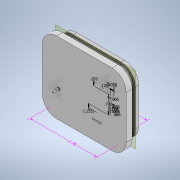
# Autodesk Inventor part: Top_Housing_K30_Elipse_O_Ring
Saved by Autodesk Inventor 2022 (Build 260153000, 153)
## iProperties
Created: 2022-06-02
Part Number: Top_Housing_K30_Elipse_O_Ring
Material: Generic
Document SubType Name: Modeling
Designer: light
Density: 1 g/cm^3
Appearance: Default
Author: light
Autodesk Inventor part; units mm, degrees
ref_plane "YZ Plane" through (0, 0, 0) normal (1, 0, 0) x (0, 1, 0)
ref_plane "XZ Plane" through (0, 0, 0) normal (0, 1, 0) x (-1, 0, 0)
ref_plane "XY Plane" through (0, 0, 0) normal (0, 0, 1) x (1, 0, 0)
sketch "Sketch1" plane through (0, 0, 0) normal (0, 0, 1) x (1, 0, 0)
  line L0 (0, 0) -> (63.246, 0)
  line L1 (63.246, 0) -> (63.246, 51.689)
  line L2 (63.246, 51.689) -> (0, 51.689)
  line L3 (0, 51.689) -> (0, 0)
  dimension "d0" = 63.246
  dimension "d1" = 51.689
  constraints: 8 end point, 2 parallel, 1 horizontal, 1 perpendicular
  measures "d0" distance of L1.end L2.end
  measures "d1" distance of L0.end L1.end
extrude "Extrusion1" add sketch "Sketch1" along normal blind 10.668
sketch "Sketch2" plane through (0, 0, 10.668) normal (0, 0, 1) x (1, 0, 0)
  line L0 (61.976, 50.6053) -> (6.35, 50.6053)
  line L1 (1.27, 45.5253) -> (1.27, 17.78)
  line L2 (6.35, 12.7) -> (61.976, 12.7)
  line L3 (61.976, 12.7) -> (61.976, 50.6053)
  arc A0 (6.35, 50.6053) -> (1.27, 45.5253) centre (6.35, 45.5253) ccw
  arc A1 (1.27, 17.78) -> (6.35, 12.7) centre (6.35, 17.78) ccw
  line L4 (0, 51.689) -> (0, 0) projected
  line L5 (63.246, 0) -> (63.246, 51.689) projected
  line L6 (0, 0) -> (63.246, 0) projected
  dimension "d4" = 5.08
  dimension "d5" = 5.08
  dimension "d6" = 1.27
  dimension "d7" = 1.27
  dimension "d8" = 60.706
  dimension "d9" = 12.7
  constraints: 8 end point, 4 point on circle, 4 tangent, 2 centre point, 2 perpendicular, 1 horizontal, 1 vertical
  measures "d4" radius of A0
  measures "d5" radius of A1
  measures "d6" distance between parallel lines of L4 L1
  measures "d7" distance between parallel lines of L5 L3
  measures "d8" distance between parallel lines of L1 L3
  measures "d9" distance between parallel lines of L6 L2
extrude "Extrusion2" cut sketch "Sketch2" against normal blind 10.668
sketch "Sketch3" plane through (0, 0, 10.668) normal (0, 0, 1) x (1, 0, 0)
  line L0 (52.451, 10.2108) -> (36.957, 10.2108)
  line L1 (36.957, 10.2108) -> (36.957, 4.1148)
  line L2 (36.957, 4.1148) -> (52.451, 4.1148)
  line L3 (52.451, 4.1148) -> (52.451, 10.2108)
  line L4 (63.246, 0) -> (63.246, 51.689) projected
  line L5 (0, 0) -> (63.246, 0) projected
  dimension "d12" = 10.795
  dimension "d13" = 15.494
  dimension "d14" = 6.096
  dimension "d15" = 4.1148
  constraints: 8 end point, 2 parallel, 1 horizontal, 1 perpendicular
  measures "d12" distance between parallel lines of L4 L3
  measures "d13" distance of L1.end L2.end
  measures "d14" distance of L0.end L1.end
  measures "d15" distance between parallel lines of L5 L2
extrude "Extrusion3" cut sketch "Sketch3" against normal blind 10.668
sketch "Sketch6" plane through (0, 0, 10.668) normal (0, 0, 1) x (1, 0, 0)
  line L0 (-3.048, 55.118) -> (67.048, 55.118) projected
  line L1 (67.048, -3.048) -> (-3.048, -3.048) projected
  line L2 (67.048, 55.118) -> (-3.048, 55.118)
  line L3 (-3.048, 55.118) -> (-3.048, -3.048)
  line L4 (-3.048, -3.048) -> (67.048, -3.048)
  line L5 (67.048, -3.048) -> (67.048, 55.118)
  line L6 (61.976, 50.6053) -> (6.35, 50.6053) projected
  line L7 (6.35, 12.7) -> (61.976, 12.7) projected
  line L8 (0, 0) -> (63.246, 0) projected
  dimension "d37" = 37.9053
  dimension "d93" = 3.048
  constraints: 8 end point, 2 parallel, 1 horizontal, 1 perpendicular
  measures "d37" distance between parallel lines of L6 L7
  measures "d93" distance between parallel lines of L1 L8
extrude "Extrusion5" add sketch "Sketch6" along normal blind 6.35
sketch "Sketch8" plane through (0, 0, 10.668) normal (0, 0, -1) x (-1, 0, 0)
  line L0 (-61.5188, 13.208) -> (-42.9768, 13.208)
  line L1 (-42.9768, 13.208) -> (-42.9768, 39.878)
  line L2 (-42.9768, 39.878) -> (-61.5188, 39.878)
  line L3 (-61.5188, 39.878) -> (-61.5188, 13.208)
  line L4 (-6.35, 12.7) -> (-61.976, 12.7) projected
  line L5 (-61.976, 12.7) -> (-61.976, 50.6053) projected
  line L6 (0, 51.689) -> (0, 0) projected
  dimension "d29" = 0.508
  dimension "d30" = 0.4572
  dimension "d31" = 18.542
  dimension "d32" = 26.67
  dimension "d33" = 42.9768
  constraints: 8 end point, 2 parallel, 1 horizontal, 1 perpendicular
  measures "d29" distance between parallel lines of L4 L0
  measures "d30" distance between parallel lines of L5 L3
  measures "d31" distance of L1.end L2.end
  measures "d32" distance of L0.end L1.end
  measures "d33" distance between parallel lines of L6 L1
extrude "Extrusion7" cut sketch "Sketch8" against normal blind 4.572
fillet "Fillet1" radius 0.254 4 edges at (52.2478, 39.878, 10.668) (42.9768, 26.543, 10.668) (52.2478, 13.208, 10.668) (61.5188, 26.543, 10.668)
sketch "Sketch9" plane through (0, 0, 15.24) normal (0, 0, -1) x (-1, 0, 0)
  line L0 (-60.2488, 17.145) -> (-57.0738, 17.145)
  line L1 (-57.0738, 17.145) -> (-57.0738, 35.941)
  line L2 (-57.0738, 35.941) -> (-60.2488, 35.941)
  line L3 (-60.2488, 35.941) -> (-60.2488, 17.145)
  line L4 (-61.5188, 13.208) -> (-61.5188, 39.878) projected
  line L5 (-61.5188, 39.878) -> (-42.9768, 39.878) projected
  line L6 (-42.9768, 13.208) -> (-61.5188, 13.208) projected
  circle A0 centre (-58.6613, 24.003) radius 0.8382
  circle A1 centre (-58.6613, 26.543) radius 0.8382
  circle A2 centre (-58.6613, 29.083) radius 0.8382
  circle A3 centre (-58.6613, 21.463) radius 0.8382
  circle A4 centre (-58.6613, 34.163) radius 0.8382
  point P0 (0, 0)
  dimension "d38" = 18.796
  dimension "d39" = 1.27
  dimension "d40" = 3.175
  dimension "d41" = 3.937
  dimension "d42" = 3.937
  dimension "d114" = 1.6764
  dimension "d116" = 1.6764
  dimension "d118" = 1.6764
  dimension "d127" = 2.54
  dimension "d128" = 2.54
  dimension "d146" = 1.6764
  dimension "d148" = 2.54
  dimension "d149" = 1.6764
  constraints: 8 end point, 5 centre point, 2 parallel, 1 horizontal, 1 perpendicular
  measures "d38" distance of L0.end L1.end
  measures "d39" distance between parallel lines of L4 L3
  measures "d40" distance of L1.end L2.end
  measures "d41" distance between parallel lines of L5 L2
  measures "d42" distance between parallel lines of L6 L0
  measures "d114" diameter of A0
  measures "d116" diameter of A1
  measures "d118" diameter of A2
  measures "d127" distance of A0.centre A1.centre
  measures "d128" distance of A1.centre A2.centre
  measures "d146" diameter of A3
  measures "d148" distance of A0.centre A3.centre
  measures "d149" diameter of A4
sketch "Sketch11" plane through (0, 0, 17.018) normal (0, 0, 1) x (1, 0, 0)
  line L0 (61.976, 12.7) -> (61.976, 50.6053) projected
  line L1 (61.976, 50.6053) -> (-0.754, 50.6053)
  line L2 (-0.754, 50.6053) -> (-0.754, 12.7)
  line L3 (-0.754, 12.7) -> (61.976, 12.7)
  line L4 (61.976, 12.7) -> (61.976, 50.6053)
  circle A0 centre (56.896, 46.8013) radius 1.0033
  circle A1 centre (4.9135, 16.5958) radius 1.0033
  point P0 (0, 0)
  dimension "d59" = 2.0066
  dimension "d60" = 2.0066
  dimension "d61" = 5.08
  constraints: 8 end point, 2 centre point, 2 parallel, 1 horizontal, 1 perpendicular
  measures "d59" diameter of A0
  measures "d60" diameter of A1
  measures "d61" distance from line of L0 A0.centre
extrude "Extrusion10" add sketch "Sketch11" along normal blind 3 contours A0 | A1
sketch "Sketch12" plane through (56.896, 46.8013, 20.018) normal (0, 0, 1) x (1, 0, 0)
  circle A0 centre (0, 0) radius 1.0033 projected
  circle A1 centre (0, 0) radius 1.2446
  point P0 (-56.896, -46.8013)
  dimension "d64" = 2.4892
  constraints: 1 centre point, 1 coincident
  measures "d64" diameter of A1
sketch "Sketch13" plane through (4.9135, 16.5958, 20.018) normal (0, 0, 1) x (1, 0, 0)
  circle A0 centre (0, 0) radius 1.2446
  point P0 (-4.9135, -16.5958)
  dimension "d65" = 2.4892
  constraints: 1 centre point
  measures "d65" diameter of A0
extrude "Extrusion11" add sketch "Sketch12" along normal blind 1 contours A0 | A1
extrude "Extrusion12" add sketch "Sketch13" along normal blind 1
sketch "Sketch14" plane through (56.896, 46.8013, 21.018) normal (0, 0, 1) x (1, 0, 0)
  circle A0 centre (0, 0) radius 0.8509
  point P0 (-56.896, -46.8013)
  dimension "d70" = 1.7018
  constraints: 1 centre point
  measures "d70" diameter of A0
sketch "Sketch15" plane through (4.9135, 16.5958, 21.018) normal (0, 0, 1) x (1, 0, 0)
  circle A0 centre (0, 0) radius 1.0033 projected
  circle A1 centre (0, 0) radius 0.8509
  point P0 (-4.9135, -16.5958)
  dimension "d71" = 1.7018
  constraints: 1 centre point, 1 coincident
  measures "d71" diameter of A1
extrude "Extrusion13" add sketch "Sketch14" along normal blind 2
extrude "Extrusion14" add sketch "Sketch15" along normal blind 2 contours A1
loft "Loft1" add section 1 edges at (4.0626, 16.5958, 23.018) section 2 edges at (3.6689, 16.5958, 21.018)
loft "Loft2" add section 1 edges at (56.0451, 46.8013, 23.018) section 2 edges at (55.6514, 46.8013, 21.018)
sketch "Sketch16" plane through (56.896, 46.8013, 23.018) normal (0, 0, 1) x (1, 0, 0)
  circle A0 centre (0, 0) radius 0.7493
  point P0 (-56.896, -46.8013)
  dimension "d84" = 1.4986
  constraints: 1 centre point
  measures "d84" diameter of A0
sketch "Sketch17" plane through (4.9135, 16.5958, 23.018) normal (0, 0, 1) x (1, 0, 0)
  circle A0 centre (0, 0) radius 0.7493
  point P0 (-4.9135, -16.5958)
  dimension "d85" = 1.4986
  constraints: 1 centre point
  measures "d85" diameter of A0
extrude "Extrusion15" cut sketch "Sketch16" against normal blind 12.446
extrude "Extrusion16" cut sketch "Sketch17" against normal blind 12.446
sketch "Sketch23" plane through (-3.048, -3.048, 10.668) normal (0, -1, 0) x (1, 0, 0)
  line L0 (70.096, 0) -> (70.096, 6.35) projected
  line L1 (0, 0) -> (70.096, 0) projected
  line L2 (70.096, 6.35) -> (0, 6.35)
  line L3 (0, 6.35) -> (0, 0)
  line L4 (0, 0) -> (70.096, 0)
  line L5 (70.096, 0) -> (70.096, 6.35)
  point P0 (3.048, -10.668)
  constraints: 8 end point, 2 parallel, 1 horizontal, 1 perpendicular
extrude "Extrusion17" add sketch "Sketch23" along normal blind 0.9525
sketch "Sketch24" plane through (-3.048, 55.118, 10.668) normal (0, 1, 0) x (1, 0, 0)
  line L0 (70.096, 0) -> (70.096, -6.35) projected
  line L1 (0, 0) -> (0, -6.35) projected
  line L2 (70.096, 0) -> (0, 0)
  line L3 (0, 0) -> (0, -6.35)
  line L4 (0, -6.35) -> (70.096, -6.35)
  line L5 (70.096, -6.35) -> (70.096, 0)
  point P0 (3.048, 10.668)
  constraints: 8 end point, 2 parallel, 1 horizontal, 1 perpendicular
extrude "Extrusion18" add sketch "Sketch24" along normal blind 0.5715
sketch "Sketch25" plane through (67.048, -4.0005, 17.018) normal (1, 0, 0) x (0, 0, -1)
  line L0 (0, 0) -> (0, 59.69) projected
  line L1 (6.35, 0) -> (6.35, 59.69) projected
  line L2 (0, 0) -> (6.35, 0)
  line L3 (6.35, 0) -> (6.35, 59.69)
  line L4 (6.35, 59.69) -> (0, 59.69)
  line L5 (0, 59.69) -> (0, 0)
  point P0 (17.018, 4.0005)
  constraints: 8 end point, 2 parallel, 1 horizontal, 1 perpendicular
extrude "Extrusion19" add sketch "Sketch25" along normal blind 0.635
sketch "Sketch26" plane through (-3.048, -4.0005, 10.668) normal (-1, 0, 0) x (0, 0, 1)
  line L0 (6.35, 0) -> (0, 0) projected
  line L1 (6.35, 0) -> (6.35, 59.69) projected
  line L2 (0, 0) -> (6.35, 0)
  line L3 (6.35, 0) -> (6.35, 59.69)
  line L4 (6.35, 59.69) -> (0, 59.69)
  line L5 (0, 59.69) -> (0, 0)
  point P0 (-10.668, 4.0005)
  constraints: 8 end point, 2 parallel, 1 horizontal, 1 perpendicular
extrude "Extrusion20" add sketch "Sketch26" along normal blind 1.397
sketch "Sketch31" plane through (0, 0, 17.018) normal (0, 0, 1) x (1, 0, 0)
  circle A0 centre (4.9135, 16.5958) radius 1.0033 projected
  circle A1 centre (4.9135, 16.5958) radius 1.27
  circle A2 centre (56.896, 46.8013) radius 0.7493 projected
  circle A3 centre (56.896, 46.8013) radius 1.27
  point P0 (0, 0)
  dimension "d102" = 2.54
  dimension "d103" = 2.54
  constraints: 2 centre point, 2 coincident
  measures "d102" diameter of A3
  measures "d103" diameter of A1
extrude "Extrusion21" add sketch "Sketch31" along normal blind 0.635
sketch "Sketch32" plane through (0, 0, 17.018) normal (0, 0, 1) x (1, 0, 0)
  circle A0 centre (4.9135, 16.5958) radius 0.7493 projected
  circle A1 centre (4.9135, 16.5958) radius 1.4749
  circle A2 centre (56.896, 46.8013) radius 1.0033 projected
  circle A3 centre (56.896, 46.8013) radius 1.4788
  point P0 (0, 0)
  constraints: 2 centre point, 2 coincident
extrude "Extrusion22" add sketch "Sketch32" along normal blind 0.381
extrude "Extrusion23" cut sketch "Sketch9" against normal blind 1.778 contours A0 | A1 | A2
sketch "Sketch33" plane through (0, 0, 10.668) normal (0, 0, -1) x (-1, 0, 0)
  circle A0 centre (-48.514, 7.493) radius 0.8382
  circle A1 centre (-45.974, 7.493) radius 0.8382
  circle A2 centre (-43.434, 7.493) radius 0.8382
  circle A3 centre (-40.894, 7.493) radius 0.8382
  line L0 (-52.451, 4.1148) -> (-52.451, 10.2108) projected
  line L1 (-36.957, 10.2108) -> (-36.957, 4.1148) projected
  line L2 (-52.451, 10.2108) -> (-36.957, 10.2108) projected
  point P0 (0, 0)
  dimension "d134" = 1.6764
  dimension "d135" = 3.937
  dimension "d136" = 1.6764
  dimension "d137" = 1.6764
  dimension "d138" = 1.6764
  dimension "d139" = 2.54
  dimension "d140" = 2.54
  dimension "d141" = 2.54
  dimension "d143" = 2.7178
  constraints: 4 centre point
  measures "d134" diameter of A0
  measures "d135" distance from line of L0 A0.centre
  measures "d136" diameter of A1
  measures "d137" diameter of A2
  measures "d138" diameter of A3
  measures "d139" distance of A1.centre A0.centre
  measures "d140" distance of A1.centre A2.centre
  measures "d141" distance of A2.centre A3.centre
  measures "d143" distance from line of L2 A0.centre
extrude "Extrusion24" cut sketch "Sketch33" against normal blind 6.35
extrude "Extrusion25" cut sketch "Sketch9" against normal blind 1.778 contours A3 | A4
sketch "Sketch39" plane through (0, 0, 10.668) normal (0, 0, -1) x (-1, 0, 0)
  line L0 (-67.683, -4.0005) -> (4.445, -4.0005) projected
  line L1 (-67.683, 55.6895) -> (4.445, 55.6895) projected
  line L2 (-67.683, -4.0005) -> (4.445, -4.0005)
  line L3 (4.445, -4.0005) -> (4.445, 55.6895)
  line L4 (4.445, 55.6895) -> (-67.683, 55.6895)
  line L5 (-67.683, 55.6895) -> (-67.683, -4.0005)
  line L6 (-75.303, -11.6205) -> (12.065, -11.6205)
  line L7 (12.065, -11.6205) -> (12.065, 63.3095)
  line L8 (12.065, 63.3095) -> (-75.303, 63.3095)
  line L9 (-75.303, 63.3095) -> (-75.303, -11.6205)
  point P0 (0, 0)
  dimension "d160" = 7.62
  dimension "d161" = 7.62
  dimension "d162" = 7.62
  dimension "d163" = 7.62
  constraints: 16 end point, 4 parallel, 2 horizontal, 2 perpendicular
  measures "d160" distance between parallel lines of L5 L9
  measures "d161" distance between parallel lines of L1 L8
  measures "d162" distance between parallel lines of L3 L7
  measures "d163" distance between parallel lines of L6 L0
extrude "Extrusion28" add sketch "Sketch39" against normal blind 6.35
sketch "Sketch41" plane through (0, 0, 10.668) normal (0, 0, -1) x (-1, 0, 0)
  line L0 (0, 0) -> (-63.246, 0) projected
  line L1 (0, 51.689) -> (0, 0) projected
  line L2 (-63.246, 0) -> (0, 0)
  line L3 (0, 0) -> (0, 51.689)
  line L4 (0, 51.689) -> (-63.246, 51.689)
  line L5 (-63.246, 51.689) -> (-63.246, 0)
  line L6 (8.128, 59.817) -> (-71.374, 59.817)
  line L7 (-71.374, 59.817) -> (-71.374, -8.128)
  line L8 (-71.374, -8.128) -> (8.128, -8.128)
  line L9 (8.128, -8.128) -> (8.128, 59.817)
  dimension "d172" = 8.128
  dimension "d173" = 8.128
  dimension "d174" = 8.128
  dimension "d175" = 8.128
  constraints: 16 end point, 4 parallel, 2 horizontal, 2 perpendicular
  measures "d172" distance between parallel lines of L5 L7
  measures "d173" distance between parallel lines of L9 L1
  measures "d174" distance between parallel lines of L4 L6
  measures "d175" distance between parallel lines of L8 L0
extrude "Extrusion30" add sketch "Sketch41" along normal blind 10.668
ref_plane "Work Plane3" through (0, 0, 5.334) normal (0, 0, -1) x (-1, 0, 0)
sketch "Sketch43" plane through (0, 0, 5.334) normal (0, 0, -1) x (-1, 0, 0)
  line L0 (-71.374, -8.128) -> (-71.374, 59.817) projected
  line L1 (-71.374, 59.817) -> (8.128, 59.817) projected
  line L2 (-71.374, -8.128) -> (8.128, -8.128)
  line L3 (8.128, -8.128) -> (8.128, 59.817)
  line L4 (8.128, 59.817) -> (-71.374, 59.817)
  line L5 (-71.374, 59.817) -> (-71.374, -8.128)
  line L6 (-56.8452, -6.2992) -> (-6.4008, -6.2992)
  line L7 (6.2992, 6.4008) -> (6.2992, 45.2882)
  line L8 (-6.4008, 57.9882) -> (-56.8452, 57.9882)
  line L9 (-69.5452, 45.2882) -> (-69.5452, 6.4008)
  arc A0 (-69.5452, 6.4008) -> (-56.8452, -6.2992) centre (-56.8452, 6.4008) ccw
  arc A1 (-56.8452, 57.9882) -> (-69.5452, 45.2882) centre (-56.8452, 45.2882) ccw
  arc A2 (6.2992, 45.2882) -> (-6.4008, 57.9882) centre (-6.4008, 45.2882) ccw
  arc A3 (-6.4008, -6.2992) -> (6.2992, 6.4008) centre (-6.4008, 6.4008) ccw
  point P0 (0, 0)
  dimension "d187" = 1.8288
  dimension "d188" = 1.8288
  dimension "d189" = 1.8288
  dimension "d190" = 1.8288
  dimension "d191" = 12.7
  constraints: 16 end point, 8 point on circle, 8 tangent, 4 centre point, 4 parallel, 3 equal radius, 2 horizontal, 2 perpendicular
  measures "d187" distance between parallel lines of L9 L0
  measures "d188" distance between parallel lines of L1 L8
  measures "d189" distance between parallel lines of L3 L7
  measures "d190" distance between parallel lines of L2 L6
  measures "d191" radius of A0
extrude "Extrusion32" cut sketch "Sketch43" along normal mid plane 3.0734
fillet "Fillet2" radius 14.732 8 edges at (71.374, 59.817, 1.8986) (71.374, 59.817, 8.7693) (-8.128, 59.817, 1.8986) (-8.128, 59.817, 8.7693) (-8.128, -8.128, 1.8986) (-8.128, -8.128, 8.7693) (71.374, -8.128, 1.8986) (71.374, -8.128, 8.7693)
fillet "Fillet3" radius 0.127 16 edges at (31.623, 59.817, 6.8707) (-3.8131, 55.5021, 6.8707) (-8.128, 25.8445, 6.8707) (-3.8131, -3.8131, 6.8707) (31.623, -8.128, 6.8707) (67.0591, -3.8131, 6.8707) (71.374, 25.8445, 6.8707) (67.0591, 55.5021, 6.8707) (71.374, 25.8445, 3.7973) (67.0591, -3.8131, 3.7973) (31.623, -8.128, 3.7973) (-3.8131, -3.8131, 3.7973) (-8.128, 25.8445, 3.7973) (-3.8131, 55.5021, 3.7973) (31.623, 59.817, 3.7973) (67.0591, 55.5021, 3.7973)
fillet "Fillet4" radius 0.254 16 edges at (65.8255, -2.5795, 6.8707) (31.623, -6.2992, 6.8707) (-2.5795, -2.5795, 6.8707) (-6.2992, 25.8445, 6.8707) (-2.5795, 54.2685, 6.8707) (31.623, 57.9882, 6.8707) (65.8255, 54.2685, 6.8707) (69.5452, 25.8445, 6.8707) (65.8255, 54.2685, 3.7973) (31.623, 57.9882, 3.7973) (-2.5795, 54.2685, 3.7973) (-6.2992, 25.8445, 3.7973) (-2.5795, -2.5795, 3.7973) (31.623, -6.2992, 3.7973) (65.8255, -2.5795, 3.7973) (69.5452, 25.8445, 3.7973)
fillet "Fillet5" radius 14.732 4 edges at (75.303, 63.3095, 13.843) (75.303, -11.6205, 13.843) (-12.065, 63.3095, 13.843) (-12.065, -11.6205, 13.843)
body "Solid1"
